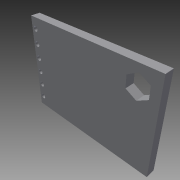
# Autodesk Inventor part: polyhexpart
Saved by Autodesk Inventor 2015 SP1 (Build 190203100, 203)
## iProperties
Created: 2015-04-18
Part Number: polyhexpart
Material: Generic
Document SubType Name: Modeling
Designer: Lab User
Density: 1 g/cm^3
Appearance: Default
Author: Lab User
Autodesk Inventor part; units mm, degrees
ref_plane "YZ Plane" through (0, 0, 0) normal (1, 0, 0) x (0, 1, 0)
ref_plane "XZ Plane" through (0, 0, 0) normal (0, 1, 0) x (-1, 0, 0)
ref_plane "XY Plane" through (0, 0, 0) normal (0, 0, 1) x (1, 0, 0)
sketch "Sketch2" plane through (0, 0, 0) normal (0, 0, 1) x (1, 0, 0)
  line L0 (-36.8686, 26.7016) -> (-30.1114, 30.7457)
  line L1 (-30.1114, 30.7457) -> (-23.2304, 26.9158)
  line L2 (-23.2304, 26.9158) -> (-23.1068, 19.0418)
  line L3 (-23.1068, 19.0418) -> (-29.864, 14.9977)
  line L4 (-29.864, 14.9977) -> (-36.7449, 18.8276)
  line L5 (-36.7449, 18.8276) -> (-36.8686, 26.7016)
  line L6 (-111.0137, 35.5717) -> (-17.2877, 35.5717)
  line L7 (-17.2877, 35.5717) -> (-17.2877, -30.4683)
  line L8 (-17.2877, -30.4683) -> (-111.0137, -30.4683)
  line L9 (-111.0137, -30.4683) -> (-111.0137, 35.5717)
  point P0 (0, 0)
  point P1 (-29.9877, 22.8717)
  dimension "d1" = 7.874
  dimension "d3" = 66.04
  dimension "d4" = 53.34
  dimension "d5" = 12.7
  dimension "d6" = 93.726
  constraints: 20 end point, 2 parallel, 1 horizontal, 1 perpendicular, 13 other
  measures "d1" vertical distance of L1.end L2.end
  measures "d3" distance of L8.end L6.start
  measures "d4" distance from line of L8 point (-29.988, 22.872)
  measures "d5" distance from line of L7 point (-29.988, 22.872)
  measures "d6" distance of L6.start L6.end
extrude "Extrusion1" add sketch "Sketch2" along normal blind 6.35
sketch "Sketch3" plane through (0, 0, 6.35) normal (0, 0, 1) x (1, 0, 0)
  circle A0 centre (-107.8387, 27.9517) radius 1.905
  line L0 (-17.2877, 35.5717) -> (-111.0137, 35.5717) projected
  line L1 (-111.0137, 35.5717) -> (-111.0137, -30.4683) projected
  circle A1 centre (-107.8387, 17.7917) radius 1.905
  circle A2 centre (-107.8387, -12.6883) radius 1.905
  circle A3 centre (-107.8387, -22.8483) radius 1.905
  line L2 (-111.0137, -30.4683) -> (-17.2877, -30.4683) projected
  circle A4 centre (-107.8387, 7.6317) radius 1.905
  circle A5 centre (-107.8387, -2.5283) radius 1.905
  point P0 (0, 0)
  dimension "d9" = 3.81
  dimension "d10" = 7.62
  dimension "d11" = 3.175
  dimension "d13" = 3.81
  dimension "d14" = 3.81
  dimension "d15" = 3.81
  dimension "d17" = 3.175
  dimension "d18" = 3.175
  dimension "d19" = 3.175
  dimension "d20" = 7.62
  dimension "d21" = 10.16
  dimension "d24" = 3.81
  dimension "d25" = 3.81
  dimension "d26" = 3.175
  dimension "d27" = 3.175
  dimension "d28" = 10.16
  dimension "d29" = 10.16
  dimension "d30" = 10.16
  dimension "d33" = 10.16
  constraints: 6 centre point
  measures "d9" diameter of A0
  measures "d10" distance from line of A0.centre L0
  measures "d11" distance from line of A0.centre L1
  measures "d13" diameter of A1
  measures "d14" diameter of A2
  measures "d15" diameter of A3
  measures "d17" distance from line of L1 A1.centre
  measures "d18" distance from line of L1 A2.centre
  measures "d19" distance from line of L1 A3.centre
  measures "d20" distance from line of L2 A3.centre
  measures "d21" distance of A3.centre A2.centre
  measures "d24" diameter of A4
  measures "d25" diameter of A5
  measures "d26" distance from line of L1 A5.centre
  measures "d27" distance from line of L1 A4.centre
  measures "d28" distance of A4.centre A1.centre
  measures "d29" distance of A4.centre A5.centre
  measures "d30" distance of A5.centre A2.centre
  measures "d33" distance of A0.centre A1.centre
extrude "Extrusion2" cut sketch "Sketch3" against normal blind 3.81
body "Solid1"
